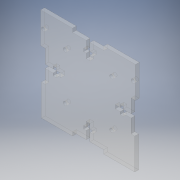
# Autodesk Inventor part: pared ateral 2
Saved by Autodesk Inventor 2016 (Build 200138000, 138)
## iProperties
Created: 2017-03-02
Part Number: pared ateral 2
Material: Generic
Document SubType Name: Modeling
Designer: jorge
Density: 1 g/cm^3
Appearance: Clear - Light
Author: jorge
## iProperties of the stored document pared ateral 2_3DPrint.ipt
Created: 2017-03-11
Part Number: pared ateral 2_3DPrint
Material: Generic
Document SubType Name: Modeling
Designer: jorge
Density: 1 g/cm^3
Appearance: Default
Author: jorge
Autodesk Inventor part; units mm, degrees
ref_plane "YZ Plane" through (0, 0, 0) normal (1, 0, 0) x (0, 1, 0)
ref_plane "XZ Plane" through (0, 0, 0) normal (0, 1, 0) x (-1, 0, 0)
ref_plane "XY Plane" through (0, 0, 0) normal (0, 0, 1) x (1, 0, 0)
sketch "Sketch1" plane through (0, 0, 0) normal (0, 0, 1) x (1, 0, 0)
  arc A0 (69, -46.7929) -> (69.7605, -47) centre (69, -48.2929) ccw projected
  line L0 (72, -47) -> (69.7605, -47) projected
  line L1 (72, -72) -> (72, -47) projected
  line L2 (47, -72) -> (72, -72) projected
  line L3 (47, -69) -> (47, -72) projected
  line L4 (22, -69) -> (33, -69) projected
  line L5 (22, -72) -> (22, -69) projected
  line L6 (-3, -72) -> (22, -72) projected
  line L7 (-3, -47) -> (-3, -72) projected
  line L8 (0, -47) -> (-3, -47) projected
  line L9 (0, -22) -> (0, -33) projected
  line L10 (-3, -22) -> (0, -22) projected
  line L11 (-3, 3) -> (-3, -8.5818) projected
  line L12 (22, 3) -> (-3, 3) projected
  line L13 (22, 0) -> (22, 3) projected
  line L14 (47, 0) -> (36, 0) projected
  line L15 (47, 3) -> (47, 0) projected
  line L16 (72, 3) -> (47, 3) projected
  line L17 (72, -22) -> (72, -9.5) projected
  line L18 (69, -22) -> (72, -22) projected
  line L19 (69, -46.7929) -> (69, -36) projected
  circle A1 centre (17, -3.5) radius 1.5 projected
  circle A2 centre (69, -16.7071) radius 1.5 projected
  circle A3 centre (20, -50.5) radius 1.5 projected
  line L20 (69.7605, -47) -> (69, -47)
  line L21 (69, -47) -> (69, -46.7929)
  line L22 (0, -36) -> (0, -47) projected
  line L23 (33, 0) -> (22, 0) projected
  line L24 (69, -33) -> (69, -22) projected
  line L25 (36, -69) -> (47, -69) projected
  line L26 (-3, -8.5818) -> (-3, -22) projected
  circle A4 centre (-1.5, -8.5818) radius 1.5 projected
  line L27 (72, -9.5) -> (72, 3) projected
  circle A5 centre (70.5, -9.5) radius 1.5 projected
  line L28 (36, -69) -> (36, -62.65) projected
  line L29 (36, -62.65) -> (38, -62.65) projected
  line L30 (38, -62.65) -> (38, -60.15) projected
  line L31 (38, -60.15) -> (36, -60.15) projected
  line L32 (36, -60.15) -> (36, -56.3) projected
  line L33 (36, -56.3) -> (33, -56.3) projected
  line L34 (33, -56.3) -> (33, -60.15) projected
  line L35 (33, -60.15) -> (31, -60.15) projected
  line L36 (31, -60.15) -> (31, -62.65) projected
  line L37 (31, -62.65) -> (33, -62.65) projected
  line L38 (33, -62.65) -> (33, -69) projected
  line L39 (0, -36) -> (6.35, -36) projected
  line L40 (6.35, -36) -> (6.35, -38) projected
  line L41 (6.35, -38) -> (8.85, -38) projected
  line L42 (8.85, -38) -> (8.85, -36) projected
  line L43 (8.85, -36) -> (12.7, -36) projected
  line L44 (12.7, -36) -> (12.7, -33) projected
  line L45 (12.7, -33) -> (8.85, -33) projected
  line L46 (8.85, -33) -> (8.85, -31) projected
  line L47 (8.85, -31) -> (6.35, -31) projected
  line L48 (6.35, -31) -> (6.35, -33) projected
  line L49 (6.35, -33) -> (0, -33) projected
  line L50 (33, 0) -> (33, -6.35) projected
  line L51 (33, -6.35) -> (31, -6.35) projected
  line L52 (31, -6.35) -> (31, -8.85) projected
  line L53 (31, -8.85) -> (33, -8.85) projected
  line L54 (33, -8.85) -> (33, -12.7) projected
  line L55 (33, -12.7) -> (36, -12.7) projected
  line L56 (36, -12.7) -> (36, -8.85) projected
  line L57 (36, -8.85) -> (38, -8.85) projected
  line L58 (38, -8.85) -> (38, -6.35) projected
  line L59 (38, -6.35) -> (36, -6.35) projected
  line L60 (36, -6.35) -> (36, 0) projected
  line L61 (69, -33) -> (62.65, -33) projected
  line L62 (62.65, -33) -> (62.65, -31) projected
  line L63 (62.65, -31) -> (60.15, -31) projected
  line L64 (60.15, -31) -> (60.15, -33) projected
  line L65 (60.15, -33) -> (56.3, -33) projected
  line L66 (56.3, -33) -> (56.3, -36) projected
  line L67 (56.3, -36) -> (60.15, -36) projected
  line L68 (60.15, -36) -> (60.15, -38) projected
  line L69 (60.15, -38) -> (62.65, -38) projected
  line L70 (62.65, -38) -> (62.65, -36) projected
  line L71 (62.65, -36) -> (69, -36) projected
  point P0 (0, 0)
  constraints: 4 end point, 1 horizontal, 1 perpendicular
extrude "Extrusion1" add sketch "Sketch1" along normal blind 3 contours L21 L20 A0 | A5 | A4 | A0 L0 L1 L2 L3 L25 L28 L29 L30 L31 L32 L33 L34 L35 L36 L37 L38 L4 L5 L6 L7 L8 L22 L39 L40 L41 L42 L43 L44 L45 L46 L47 L48 L49 L9 L10 L26 L11 L12 L13 L23 L50 L51 L52 L53 L54 L55 L56 L57 L58 L59 L60 L14 L15 L16 L27 L17 L18 L24 L61 L62 L63 L64 L65 L66 L67 L68 L69 L70 L71 L19 | A1 | A2 | A3
sketch "Sketch2" plane through (0, 0, 3) normal (0, 0, 1) x (1, 0, 0)
  circle A0 centre (16, -15.05) radius 1.5 projected
  circle A1 centre (53.3, -15.05) radius 1.5 projected
  circle A2 centre (16, -52.35) radius 1.5 projected
  circle A3 centre (53.3, -52.35) radius 1.5 projected
  point P0 (0, 0)
extrude "Extrusion2" cut sketch "Sketch2" against normal blind 3
sketch "Sketch3" plane through (0, 0, 3) normal (0, 0, 1) x (1, 0, 0)
  line L0 (22, 3) -> (-3, 3) projected
  circle A0 centre (16, -52.35) radius 1.5 projected
  circle A1 centre (16, -15.05) radius 1.5 projected
  circle A2 centre (53.3, -15.05) radius 1.5 projected
  circle A3 centre (53.3, -52.35) radius 1.5 projected
  line L1 (72, -47) -> (69, -47) projected
  line L2 (69, -47) -> (69, -36) projected
  line L3 (69, -22) -> (72, -22) projected
  line L4 (72, -22) -> (72, 3) projected
  line L5 (72, 3) -> (47, 3) projected
  line L6 (47, 3) -> (47, 0) projected
  line L7 (47, 0) -> (36, 0) projected
  line L8 (22, 0) -> (22, 3) projected
  line L9 (22, 3) -> (-3, 3) projected
  line L10 (-3, 3) -> (-3, -22) projected
  line L11 (-3, -22) -> (0, -22) projected
  line L12 (0, -22) -> (0, -33) projected
  line L13 (0, -47) -> (-3, -47) projected
  line L14 (-3, -47) -> (-3, -72) projected
  line L15 (-3, -72) -> (22, -72) projected
  line L16 (22, -72) -> (22, -69) projected
  line L17 (22, -69) -> (33, -69) projected
  line L18 (47, -69) -> (47, -72) projected
  line L19 (47, -72) -> (72, -72) projected
  line L20 (72, -72) -> (72, -47) projected
  line L21 (47, 0) -> (22, 0) projected
  line L22 (34.5, 0) -> (34.5, -12.7)
  line L23 (34.5, -6.35) -> (31, -6.35)
  line L24 (31, -6.35) -> (31, -8.85)
  line L25 (31, -8.85) -> (38, -8.85)
  line L26 (38, -8.85) -> (38, -6.35)
  line L27 (38, -6.35) -> (34.5, -6.35)
  line L28 (34.5, -12.7) -> (36, -12.7)
  line L29 (36, -12.7) -> (36, 0)
  line L30 (34.5, -12.7) -> (33, -12.7)
  line L31 (33, -12.7) -> (33, 0)
  line L32 (33, 0) -> (36, 0)
  line L33 (0, -22) -> (0, -47) projected
  line L34 (0, -34.5) -> (12.7, -34.5)
  line L35 (6.35, -34.5) -> (6.35, -31)
  line L36 (6.35, -31) -> (8.85, -31)
  line L37 (8.85, -31) -> (8.85, -38)
  line L38 (8.85, -38) -> (6.35, -38)
  line L39 (6.35, -38) -> (6.35, -34.5)
  line L40 (12.7, -34.5) -> (12.7, -36)
  line L41 (12.7, -36) -> (12.7, -33)
  line L42 (12.7, -33) -> (0, -33)
  line L43 (0, -36) -> (0, -33)
  line L44 (0, -36) -> (12.7, -36)
  line L45 (69, -34.5) -> (56.3, -34.5)
  line L46 (62.65, -34.5) -> (62.65, -31)
  line L47 (62.65, -31) -> (60.15, -31)
  line L48 (60.15, -31) -> (60.15, -38)
  line L49 (60.15, -38) -> (62.65, -38)
  line L50 (56.3, -34.5) -> (56.3, -36)
  line L51 (56.3, -36) -> (56.3, -33)
  line L52 (56.3, -33) -> (69, -33)
  line L53 (69, -36) -> (69, -33)
  line L54 (69, -36) -> (56.3, -36)
  line L55 (47, -69) -> (22, -69)
  line L56 (47, -69) -> (22, -69)
  line L57 (34.5, -69) -> (34.5, -56.3)
  line L58 (34.5, -62.65) -> (31, -62.65)
  line L59 (31, -62.65) -> (31, -60.15)
  line L60 (31, -60.15) -> (38, -60.15)
  line L61 (38, -60.15) -> (38, -62.65)
  line L62 (38, -62.65) -> (34.5, -62.65)
  line L63 (34.5, -56.3) -> (36, -56.3)
  line L64 (36, -56.3) -> (36, -69)
  line L65 (34.5, -56.3) -> (33, -56.3)
  line L66 (33, -56.3) -> (33, -69)
  line L67 (33, -69) -> (36, -69)
  line L68 (0, -33) -> (12.7, -33)
  line L69 (12.7, -33) -> (12.7, -36)
  line L70 (12.7, -36) -> (0, -36)
  line L71 (0, -36) -> (0, -33)
  line L72 (33, 0) -> (36, 0)
  line L73 (36, 0) -> (36, -12.7)
  line L74 (36, -12.7) -> (33, -12.7)
  line L75 (33, -12.7) -> (33, 0)
  line L76 (56.3, -33) -> (69, -33)
  line L77 (69, -33) -> (69, -36)
  line L78 (69, -36) -> (56.3, -36)
  line L79 (56.3, -36) -> (56.3, -33)
  line L80 (33, -56.3) -> (36, -56.3)
  line L81 (36, -56.3) -> (36, -69)
  line L82 (36, -69) -> (33, -69)
  line L83 (33, -69) -> (33, -56.3)
  line L84 (60.15, -38) -> (62.65, -38)
  line L85 (62.65, -38) -> (62.65, -31)
  line L86 (62.65, -31) -> (60.15, -31)
  line L87 (60.15, -31) -> (60.15, -38)
  line L88 (69, -33) -> (69, -22) projected
  line L89 (33, 0) -> (22, 0) projected
  line L90 (0, -36) -> (0, -47) projected
  line L91 (36, -69) -> (47, -69) projected
  line L92 (69, -36) -> (62.65, -36) projected
  line L93 (62.65, -36) -> (62.65, -38) projected
  line L94 (62.65, -38) -> (60.15, -38) projected
  line L95 (60.15, -38) -> (60.15, -36) projected
  line L96 (60.15, -36) -> (56.3, -36) projected
  line L97 (56.3, -36) -> (56.3, -33) projected
  line L98 (56.3, -33) -> (60.15, -33) projected
  line L99 (60.15, -33) -> (60.15, -31) projected
  line L100 (60.15, -31) -> (62.65, -31) projected
  line L101 (62.65, -31) -> (62.65, -33) projected
  line L102 (62.65, -33) -> (69, -33) projected
  line L103 (36, 0) -> (36, -6.35) projected
  line L104 (36, -6.35) -> (38, -6.35) projected
  line L105 (38, -6.35) -> (38, -8.85) projected
  line L106 (38, -8.85) -> (36, -8.85) projected
  line L107 (36, -8.85) -> (36, -12.7) projected
  line L108 (36, -12.7) -> (33, -12.7) projected
  line L109 (33, -12.7) -> (33, -8.85) projected
  line L110 (33, -8.85) -> (31, -8.85) projected
  line L111 (31, -8.85) -> (31, -6.35) projected
  line L112 (31, -6.35) -> (33, -6.35) projected
  line L113 (33, -6.35) -> (33, 0) projected
  line L114 (0, -33) -> (6.35, -33) projected
  line L115 (6.35, -33) -> (6.35, -31) projected
  line L116 (6.35, -31) -> (8.85, -31) projected
  line L117 (8.85, -31) -> (8.85, -33) projected
  line L118 (8.85, -33) -> (12.7, -33) projected
  line L119 (12.7, -33) -> (12.7, -36) projected
  line L120 (12.7, -36) -> (8.85, -36) projected
  line L121 (8.85, -36) -> (8.85, -38) projected
  line L122 (8.85, -38) -> (6.35, -38) projected
  line L123 (6.35, -38) -> (6.35, -36) projected
  line L124 (6.35, -36) -> (0, -36) projected
  line L125 (33, -69) -> (33, -62.65) projected
  line L126 (33, -62.65) -> (31, -62.65) projected
  line L127 (31, -62.65) -> (31, -60.15) projected
  line L128 (31, -60.15) -> (33, -60.15) projected
  line L129 (33, -60.15) -> (33, -56.3) projected
  line L130 (33, -56.3) -> (36, -56.3) projected
  line L131 (36, -56.3) -> (36, -60.15) projected
  line L132 (36, -60.15) -> (38, -60.15) projected
  line L133 (38, -60.15) -> (38, -62.65) projected
  line L134 (38, -62.65) -> (36, -62.65) projected
  line L135 (36, -62.65) -> (36, -69) projected
  point P0 (0, 0)
  dimension "d4" = 12.7
  dimension "d5" = 3.5
  dimension "d6" = 2.5
  dimension "d7" = 7
  dimension "d8" = 1.5
  dimension "d9" = 1.5
  dimension "d10" = 12.7
  dimension "d11" = 3.5
  dimension "d12" = 2.5
  dimension "d13" = 7
  dimension "d14" = 1.5
  dimension "d15" = 3
  constraints: 130 end point, 22 symmetric about line, 18 perpendicular, 12 parallel, 12 point on line, 8 horizontal, 4 midpoint, 2 vertical, 1 collinear
  measures "d4" distance of L22.start L22.end
  measures "d5" distance of L23.start L23.end
  measures "d6" distance of L23.end L24.end
  measures "d7" distance of L24.end L25.end
  measures "d8" distance of L22.end L28.end
  measures "d9" distance of L22.end L30.end
  measures "d10" distance of L34.start L34.end
  measures "d11" distance of L35.start L35.end
  measures "d12" distance of L35.end L36.end
  measures "d13" distance of L36.end L37.end
  measures "d14" distance of L34.end L40.end
  measures "d15" distance of L40.end L41.end
extrude "Extrusion3" cut sketch "Sketch3" against normal blind 25.4 contours L21 L22 L23 L31 | L21 L29 L27 L22 | L31 L25 L24 L23 | L23 L22 L25 L31 | L42 L35 L34 L33 | L27 L29 L25 L22 | L25 L22 L30 L31 | L34 L39 L44 L33 | L42 L37 L34 L35 | L35 L36 L37 L42 | L27 L26 L25 L29 | L25 L29 L28 L22 | L34 L37 L44 L39 | L42 L41 L34 L37 | L44 L37 L38 L39 | L34 L40 L44 L37 | L53 L45 L46 L52 | L52 L48 L47 L46 | L46 L45 L48 L52 | L53 L54 L85 L45 | L66 L58 L57 L55 | L85 L54 L48 L45 | L48 L45 L51 L52 | L57 L62 L64 L55 | L66 L60 L57 L58 | L58 L59 L60 L66 | L48 L54 L50 L45 | L85 L49 L48 L54 | L57 L60 L64 L62 | L66 L65 L57 L60 | L64 L60 L61 L62 | L57 L63 L64 L60
sketch "Sketch4" plane through (0, 0, 3) normal (0, 0, 1) x (1, 0, 0)
  line L0 (-3, -11) -> (-3, -8) projected
  line L1 (-3, 3) -> (-3, -22) projected
  line L2 (-3, -9.5) -> (-1.5, -9.5)
  line L3 (72, -22) -> (72, 3) projected
  line L4 (72, -9.5) -> (70.5, -9.5)
  circle A0 centre (70.5, -9.5) radius 1.5
  circle A1 centre (-1.5, -9.5) radius 1.5
  point P0 (0, 0)
  dimension "d18" = 1.5
  dimension "d19" = 1.5
  constraints: 4 end point, 2 coincident, 2 horizontal, 2 horizontal alignment, 2 midpoint, 4 other
  measures "d18" distance of L2.start L2.end
  measures "d19" distance of L4.start L4.end
extrude "Extrusion4" cut sketch "Sketch4" against normal blind 25.4
sketch "Sketch5" plane through (72, 3, 3) normal (1, 0, 0) x (0, 0, -1)
  line L0 (0, -12.5) -> (3, -12.5) projected
  line L1 (3, -12.5) -> (3, 0) projected
  line L2 (3, 0) -> (0, 0) projected
  line L3 (0, -12.5) -> (0, 0) projected
  line L4 (0, -25) -> (0, -12.5) projected
  line L5 (3, -25) -> (0, -25) projected
  line L6 (3, -25) -> (3, -12.5) projected
  point P0 (3, -3)
extrude "Extrusion5" add sketch "Sketch5" along normal blind 0.5
sketch "Sketch6" plane through (-3, 3, 0) normal (-1, 0, 0) x (0, 0, 1)
  line L0 (3, -12.5) -> (0, -12.5) projected
  line L1 (3, 0) -> (3, -12.5) projected
  line L2 (0, 0) -> (3, 0) projected
  line L3 (0, 0) -> (0, -12.5) projected
  line L4 (0, -12.5) -> (0, -25) projected
  line L5 (0, -25) -> (3, -25) projected
  line L6 (3, -12.5) -> (3, -25) projected
  line L7 (3, -12.5) -> (0, -12.5) projected
  line L8 (0, -12.5) -> (0, -25) projected
  line L9 (0, -25) -> (3, -25) projected
  line L10 (3, -12.5) -> (3, -25) projected
  line L11 (3, 0) -> (3, -12.5) projected
  line L12 (0, 0) -> (3, 0) projected
  line L13 (0, 0) -> (0, -12.5) projected
  point P0 (0, -3)
extrude "Extrusion6" add sketch "Sketch6" along normal blind 0.5
body "Solid1"
